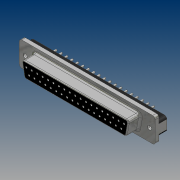
# Autodesk Inventor part: DB37-_0_6960_J
Saved by Autodesk Inventor 2012 (Build 160160000, 160)
## iProperties
Company: Team 801
Created: 2007-09-01
Part Number: DB37-_0_6960_J
Document SubType Name: Modeling
Designer: Jeffrey M
Mass: 6.17008 g
Surface Area: 43.5533 cm^2
Volume: 6.17008 cm^3
Density: 1 g/cm^3
Catalog Web Link: www.team801.org
Material: Default
Author: Jeffrey M
Autodesk Inventor part; units mm, degrees
ref_plane "YZ Plane" through (0, 0, 0) normal (1, 0, 0) x (0, 1, 0)
ref_plane "XZ Plane" through (0, 0, 0) normal (0, 1, 0) x (-1, 0, 0)
ref_plane "XY Plane" through (0, 0, 0) normal (0, 0, 1) x (1, 0, 0)
sketch "Sketch1" plane through (0, 0, 0) normal (0, 0, 1) x (1, 0, 0)
  line L0 (0, 9.1532) -> (0, -9.1532) construction
  line L1 (-48.9412, 0) -> (48.9412, 0) construction
  line L2 (-33.425, 6.275) -> (33.425, 6.275)
  line L3 (34.695, 5.005) -> (34.695, -5.005)
  line L4 (33.425, -6.275) -> (-33.425, -6.275)
  line L5 (-34.695, -5.005) -> (-34.695, 5.005)
  arc A0 (-33.425, 6.275) -> (-34.695, 5.005) centre (-33.425, 5.005) ccw
  arc A1 (-34.695, -5.005) -> (-33.425, -6.275) centre (-33.425, -5.005) ccw
  arc A2 (33.425, -6.275) -> (34.695, -5.005) centre (33.425, -5.005) ccw
  arc A3 (34.695, 5.005) -> (33.425, 6.275) centre (33.425, 5.005) ccw
  point P0 (-34.695, 6.275)
  point P1 (34.695, -6.275)
  point P2 (34.695, 6.275)
  point P3 (-34.695, -6.275)
  dimension "d0" = 69.39
  dimension "d1" = 12.55
  dimension "d6" = 1.27
  constraints: 8 end point, 8 point on circle, 8 point on line, 8 tangent, 4 centre point, 3 equal radius, 2 parallel, 1 horizontal, 1 perpendicular, 2 other
  measures "d0" distance of point (-34.695, 6.275) point (34.695, 6.275)
  measures "d1" distance of point (-34.695, -6.275) point (-34.695, 6.275)
  measures "d6" radius of A0
extrude "Base Flange" add sketch "Sketch1" along normal mid plane 1.91
sketch "Sketch2" plane through (0, 0, 0.955) normal (0, 0, 1) x (1, 0, 0)
  line L0 (34.695, 5.005) -> (34.695, -5.005) projected
  line L1 (-27.1572, 2.4595) -> (-26.2121, -2.9005)
  line L2 (-24.9614, -3.95) -> (24.9614, -3.95)
  line L3 (26.2121, -2.9005) -> (27.1572, 2.4595)
  line L4 (25.9065, 3.95) -> (-25.9065, 3.95)
  line L5 (-48.573, 0) -> (48.573, 0) construction
  line L6 (0, 8.785) -> (0, -8.785) construction
  arc A0 (-25.9065, 3.95) -> (-27.1572, 2.4595) centre (-25.9065, 2.68) ccw
  arc A1 (-26.2121, -2.9005) -> (-24.9614, -3.95) centre (-24.9614, -2.68) ccw
  arc A2 (24.9614, -3.95) -> (26.2121, -2.9005) centre (24.9614, -2.68) ccw
  arc A3 (27.1572, 2.4595) -> (25.9065, 3.95) centre (25.9065, 2.68) ccw
  point P0 (-27.42, 3.95)
  point P1 (27.42, 3.95)
  dimension "d7" = 7.9
  dimension "d8" = 54.84
  dimension "d9" = 10
  dimension "d10" = 1.27
  constraints: 8 end point, 8 point on circle, 8 tangent, 4 centre point, 4 point on line, 3 equal radius, 1 parallel, 1 perpendicular, 2 other
  measures "d7" distance between parallel lines of L4 L2
  measures "d8" distance of point (-27.42, 3.95) point (27.42, 3.95)
  measures "d9" angle of L6 L1
  measures "d10" radius of A0
extrude "Socket Side Boss Housing" add sketch "Sketch2" along normal blind 6.17
sketch "Sketch3" plane through (0, 0, -0.955) normal (0, 0, -1) x (-1, 0, 0)
  line L0 (-33.425, 3.55) -> (33.425, 3.55)
  line L1 (34.695, 2.28) -> (34.695, -2.28)
  line L2 (33.425, -3.55) -> (-33.425, -3.55)
  line L3 (-34.695, -2.28) -> (-34.695, 2.28)
  line L4 (0, -8.785) -> (0, 8.785) construction
  line L5 (-48.9412, 0) -> (48.9412, 0) construction
  arc A0 (-33.425, 3.55) -> (-34.695, 2.28) centre (-33.425, 2.28) ccw
  arc A1 (-34.695, -2.28) -> (-33.425, -3.55) centre (-33.425, -2.28) ccw
  arc A2 (33.425, -3.55) -> (34.695, -2.28) centre (33.425, -2.28) ccw
  arc A3 (34.695, 2.28) -> (33.425, 3.55) centre (33.425, 2.28) ccw
  line L6 (-34.695, -5.005) -> (-34.695, 5.005) construction
  point P0 (-34.695, 3.55)
  point P1 (34.695, 3.55)
  point P2 (-34.695, -3.55)
  dimension "d13" = 7.1
  dimension "d15" = 1.27
  constraints: 8 end point, 8 point on circle, 8 tangent, 7 point on line, 4 centre point, 3 equal radius, 2 parallel, 1 horizontal, 1 perpendicular, 2 other
  measures "d13" distance of point (-34.695, -3.55) point (-34.695, 3.55)
  measures "d15" radius of A0
extrude "Board Side Plastic Boss" add sketch "Sketch3" along normal blind 4.08
sketch "Sketch7" plane through (0, 0, 0.955) normal (0, 0, 1) x (1, 0, 0)
  line L0 (0, 9.1532) -> (0, -9.1532) projected
  line L1 (-48.9412, 0) -> (48.9412, 0) construction
  point P0 (0, 0)
  point P1 (-31.75, 0)
  point P2 (31.75, 0)
  dimension "d39" = 63.5
  constraints: 1 point on line, 1 symmetric about line
  measures "d39" diameter of point (-31.75, 0) L0
hole "Hole1" at (-31.75, 0, 0.955) at (31.75, 0, 0.955) direction (0, 0, -1) diameter 2.156 end through all thread size "4-40 UNC" class "2B" standard "ANSI Unified Screw Threads"
sketch "Sketch5" plane through (0, 0, -5.035) normal (0, 0, -1) x (-1, 0, 0)
  circle A0 centre (-24.93, 1.42) radius 0.4445
  circle A1 centre (-23.545, -1.42) radius 0.4445
  line L0 (-48.573, 0) -> (48.573, 0) construction
  line L1 (0, -8.785) -> (0, 8.785) construction
  circle A2 centre (-22.16, 1.42) radius 0.4445
  dimension "d23" = 2.84
  dimension "d25" = 0.889
  dimension "d26" = 2.77
  dimension "d27" = 1.385
  dimension "d28" = 1.42
  dimension "d29" = 24.93
  constraints: 3 centre point, 2 equal radius, 1 horizontal alignment
  measures "d23" vertical distance of A1.centre A0.centre
  measures "d25" diameter of A1
  measures "d26" distance of A2.centre A0.centre
  measures "d27" horizontal distance of A1.centre A0.centre
  measures "d28" distance from line of A0.centre L0
  measures "d29" distance from line of L1 A0.centre
extrude "Pin Extrusion" add sketch "Sketch5" along normal blind 3.18
sketch "Sketch6" plane through (0, 0, 7.125) normal (0, 0, 1) x (1, 0, 0)
  circle A0 centre (24.93, 1.42) radius 0.4445 projected
  circle A1 centre (23.545, -1.42) radius 0.4445 projected
  circle A2 centre (22.16, 1.42) radius 0.4445 projected
extrude "Socket Cut" cut sketch "Sketch6" against normal blind 6.1
pattern_linear "Pin and Hole Pattern" count 18 spacing 2.77 along (-1, 0, 0) of "Pin Extrusion", "Socket Cut"
fillet "Fillets" radius 1 8 edges at (0, 3.95, 0.955) (26.8793, 3.4963, 0.955) (26.6846, -0.2205, 0.955) (25.7777, -3.6529, 0.955) (0, -3.95, 0.955) (-25.7777, -3.6529, 0.955) (-26.6846, -0.2205, 0.955) (-26.8793, 3.4963, 0.955)
fillet "Fillets" radius 0.5 8 edges at (0, -3.95, 7.125) (-25.7777, -3.6529, 7.125) (-26.6846, -0.2205, 7.125) (-26.8793, 3.4963, 7.125) (0, 3.95, 7.125) (26.8793, 3.4963, 7.125) (26.6846, -0.2205, 7.125) (25.7777, -3.6529, 7.125)
equation "\"d27\" = 0.5 * d26"
equation "\"d28\" = 0.5 * d23"
equation "\"d29\" = 9 * d26"
equation "\"d36\" = d26"
body "Solid1"
